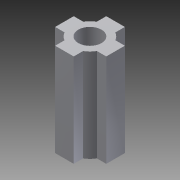
# Autodesk Inventor part: motor_axis_cross_2.5
Saved by Autodesk Inventor 2015 (Build 190159000, 159)
## iProperties
Created: 2016-05-30
Part Number: motor_axis_cross_2.5
Material: Plástico ABS
Document SubType Name: Modeling
Designer: JavierPC
Density: 1.06 g/cm^3
Appearance: Suave - Blanco
Author: Javier Pérez de Frutos
Title: Adaptador para el eje del motor
Autodesk Inventor part; units mm, degrees
ref_plane "YZ Plane" through (0, 0, 0) normal (1, 0, 0) x (0, 1, 0)
ref_plane "XZ Plane" through (0, 0, 0) normal (0, 1, 0) x (-1, 0, 0)
sketch "Boceto3" plane through (0, 0, 0) normal (0, 0, 1) x (1, 0, 0)
  circle A0 centre (0, 0) radius 2
  dimension "d13" = 4
  constraints: 1 centre point, 1 coincident
  measures "d13" diameter of A0
sketch "Boceto1" plane through (0, 0, 0) normal (0, 0, 1) x (1, 0, 0)
  line L0 (-1, 2.7591) -> (1, 2.7591)
  line L1 (1, 2.7591) -> (1, -2.7409)
  line L2 (1, -2.7409) -> (-1, -2.7409)
  line L3 (-1, -2.7409) -> (-1, 2.7591)
  line L4 (0, 5.941) -> (0, -7.9228)
  line L5 (-6.4273, 0.0091) -> (13.1091, 0.0091)
  line L6 (-2.75, 1.0091) -> (2.75, 1.0091)
  line L7 (2.75, 1.0091) -> (2.75, -0.9909)
  line L8 (2.75, -0.9909) -> (-2.75, -0.9909)
  line L9 (-2.75, -0.9909) -> (-2.75, 1.0091)
  point P0 (0, 0)
  point P1 (0, 2.7591)
  point P2 (1, 0.0091)
  point P3 (-2.75, 0.0091)
  point P4 (0, -0.9909)
  dimension "d0" = 2
  dimension "d1" = 5.5
  dimension "d2" = 5.5
  dimension "d3" = 2
  constraints: 20 end point, 5 midpoint, 4 horizontal, 4 parallel, 3 point on line, 2 perpendicular, 2 vertical
  measures "d0" distance of L1.end L2.end
  measures "d1" distance of L0.end L1.end
  measures "d2" distance of L7.end L8.end
  measures "d3" distance of L6.end L7.end
ref_plane "Plano de trabajo1" through (0, 0, 11) normal (0, 0, 1) x (1, 0, 0)
extrude "Extrusión2" add sketch "Boceto1" along normal blind 10
extrude "Extrusión3" add sketch "Boceto3" along normal blind 10
sketch "Boceto2" plane through (0, 0, 10) normal (0, 0, 1) x (1, 0, 0)
  point P0 (0, 0)
  point P1 (0, 0)
  constraints: 1 coincident
hole "Agujero1" at (0, 0, 10) direction (0, 0, -1) diameter 2.5 end through all
